Autodesk Inventor part; units mm, degrees
(part 3 of 4)
  line L1325 (-59.5167, -62.4834) -> (-59.6659, -62.6191)
  line L1326 (-59.6659, -62.6191) -> (-59.8276, -62.74)
  line L1327 (-59.8276, -62.74) -> (-60.0007, -62.8451)
  line L1328 (-60.0007, -62.8451) -> (-60.1844, -62.9336)
  line L1329 (-60.1844, -62.9336) -> (-60.3773, -63.0039)
  line L1330 (-60.3773, -63.0039) -> (-60.5785, -63.0559)
  line L1331 (-60.5785, -63.0559) -> (-60.7869, -63.0876)
  line L1332 (-60.7869, -63.0876) -> (-61.0017, -63.0986)
  line L1333 (-61.0017, -63.0986) -> (-61.2163, -63.0876)
  line L1334 (-61.2163, -63.0876) -> (-61.4249, -63.0559)
  line L1335 (-61.4249, -63.0559) -> (-61.6261, -63.0039)
  line L1336 (-61.6261, -63.0039) -> (-61.8191, -62.9336)
  line L1337 (-61.8191, -62.9336) -> (-62.0027, -62.8451)
  line L1338 (-62.0027, -62.8451) -> (-62.1758, -62.74)
  line L1339 (-62.1758, -62.74) -> (-62.3375, -62.6191)
  line L1340 (-62.3375, -62.6191) -> (-62.4865, -62.4834)
  line L1341 (-62.4865, -62.4834) -> (-62.6221, -62.3342)
  line L1342 (-62.6221, -62.3342) -> (-62.743, -62.1726)
  line L1343 (-62.743, -62.1726) -> (-62.8483, -61.9993)
  line L1344 (-62.8483, -61.9993) -> (-62.9366, -61.816)
  line L1345 (-62.9366, -61.816) -> (-63.0073, -61.6231)
  line L1346 (-63.0073, -61.6231) -> (-63.0589, -61.4216)
  line L1347 (-63.0589, -61.4216) -> (-63.0908, -61.2131)
  line L1348 (-63.0908, -61.2131) -> (-63.1017, -60.9985)
  line L1349 (59.4388, -47.6026) -> (59.4468, -47.4441)
  line L1350 (59.4468, -47.4441) -> (59.4705, -47.2901)
  line L1351 (59.4705, -47.2901) -> (59.5088, -47.1417)
  line L1352 (59.5088, -47.1417) -> (59.5608, -46.999)
  line L1353 (59.5608, -46.999) -> (59.7038, -46.7358)
  line L1354 (59.7038, -46.7358) -> (59.8929, -46.5064)
  line L1355 (59.8929, -46.5064) -> (60.1223, -46.3172)
  line L1356 (60.1223, -46.3172) -> (60.3855, -46.1743)
  line L1357 (60.3855, -46.1743) -> (60.5278, -46.1222)
  line L1358 (60.5278, -46.1222) -> (60.6767, -46.084)
  line L1359 (60.6767, -46.084) -> (60.8303, -46.0606)
  line L1360 (60.8303, -46.0606) -> (60.9888, -46.0527)
  line L1361 (60.9888, -46.0527) -> (61.1473, -46.0606)
  line L1362 (61.1473, -46.0606) -> (61.3013, -46.084)
  line L1363 (61.3013, -46.084) -> (61.4497, -46.1222)
  line L1364 (61.4497, -46.1222) -> (61.5924, -46.1743)
  line L1365 (61.5924, -46.1743) -> (61.8556, -46.3172)
  line L1366 (61.8556, -46.3172) -> (62.085, -46.5064)
  line L1367 (62.085, -46.5064) -> (62.2741, -46.7358)
  line L1368 (62.2741, -46.7358) -> (62.4171, -46.999)
  line L1369 (62.4171, -46.999) -> (62.4691, -47.1417)
  line L1370 (62.4691, -47.1417) -> (62.5074, -47.2901)
  line L1371 (62.5074, -47.2901) -> (62.5308, -47.4441)
  line L1372 (62.5308, -47.4441) -> (62.5391, -47.6026)
  line L1373 (62.5391, -47.6026) -> (62.5308, -47.7611)
  line L1374 (62.5308, -47.7611) -> (62.5074, -47.9147)
  line L1375 (62.5074, -47.9147) -> (62.4691, -48.0636)
  line L1376 (62.4691, -48.0636) -> (62.4171, -48.2058)
  line L1377 (62.4171, -48.2058) -> (62.2741, -48.469)
  line L1378 (62.2741, -48.469) -> (62.085, -48.6985)
  line L1379 (62.085, -48.6985) -> (61.8556, -48.888)
  line L1380 (61.8556, -48.888) -> (61.5924, -49.0306)
  line L1381 (61.5924, -49.0306) -> (61.4497, -49.083)
  line L1382 (61.4497, -49.083) -> (61.3013, -49.1209)
  line L1383 (61.3013, -49.1209) -> (61.1473, -49.1446)
  line L1384 (61.1473, -49.1446) -> (60.9888, -49.1526)
  line L1385 (60.9888, -49.1526) -> (60.8303, -49.1446)
  line L1386 (60.8303, -49.1446) -> (60.6767, -49.1209)
  line L1387 (60.6767, -49.1209) -> (60.5278, -49.083)
  line L1388 (60.5278, -49.083) -> (60.3855, -49.0306)
  line L1389 (60.3855, -49.0306) -> (60.1223, -48.888)
  line L1390 (60.1223, -48.888) -> (59.8929, -48.6985)
  line L1391 (59.8929, -48.6985) -> (59.7038, -48.469)
  line L1392 (59.7038, -48.469) -> (59.5608, -48.2058)
  line L1393 (59.5608, -48.2058) -> (59.5088, -48.0636)
  line L1394 (59.5088, -48.0636) -> (59.4705, -47.9147)
  line L1395 (59.4705, -47.9147) -> (59.4468, -47.7611)
  line L1396 (59.4468, -47.7611) -> (59.4388, -47.6026)
  line L1397 (-2.0682, 0) -> (2.0682, 0) construction
  line L1398 (0, 4.1364) -> (0, -4.1364) construction
  point P0 (0, 0)
  point P1 (0, 0)
  constraints: 1814 end point, 5 midpoint, 492 other
sketch "Sketch3" plane through (0, 0, 0) normal (0, 1, 0) x (-1, 0, 0)
  line L0 (-71.8987, -44.9902) -> (-71.8987, 45.0005) construction
  line L1 (71.8915, 29.9989) -> (71.8915, -29.9985) construction
  line L2 (-51.3449, 71.9911) -> (51.3515, 71.9911) construction
  line L3 (51.348, -71.9835) -> (-51.3468, -71.9835) construction
  line L4 (61.9413, 71.941) -> (-61.9413, 71.941)
  line L5 (-71.9413, 61.941) -> (-71.9413, -61.941)
  line L6 (-61.9413, -71.941) -> (61.9413, -71.941)
  line L7 (71.9413, -61.941) -> (71.9413, 61.941)
  line L8 (71.9413, 71.941) -> (-71.9413, -71.941) construction
  line L9 (-71.9413, 71.941) -> (71.9413, -71.941) construction
  arc A0 (-61.9413, 71.941) -> (-71.9413, 61.941) centre (-61.9413, 61.941) ccw
  arc A1 (71.9413, 61.941) -> (61.9413, 71.941) centre (61.9413, 61.941) ccw
  arc A2 (61.9413, -71.941) -> (71.9413, -61.941) centre (61.9413, -61.941) ccw
  arc A3 (-71.9413, -61.941) -> (-61.9413, -71.941) centre (-61.9413, -61.941) ccw
  line L10 (-41.1674, 56.1487) -> (-3.9986, 18.9801)
  line L11 (-3.9986, 18.9801) -> (-3.9986, 56.1578)
  line L12 (-3.9986, 56.1578) -> (-41.1674, 56.1487)
  line L13 (4.0012, 56.1578) -> (41.1357, 56.1578)
  line L14 (41.1357, 56.1578) -> (4.0012, 19.0231)
  line L15 (4.0012, 19.0231) -> (4.0012, 56.1578)
  line L16 (19.3996, 4.4418) -> (19.3996, -4.4032)
  line L17 (19.3996, -4.4032) -> (50.0055, -35.0091)
  line L18 (50.0055, -35.0091) -> (50.0055, 35.0476)
  line L19 (50.0055, 35.0476) -> (19.3996, 4.4418)
  line L20 (41.1109, -56.0179) -> (4.0012, -18.9084)
  line L21 (4.0012, -18.9084) -> (4.0012, -56.0179)
  line L22 (4.0012, -56.0179) -> (41.1109, -56.0179)
  line L23 (-3.9986, -56.0179) -> (-41.1514, -56.0179)
  line L24 (-41.1514, -56.0179) -> (-3.9986, -18.8653)
  line L25 (-3.9986, -18.8653) -> (-3.9986, -56.0179)
  line L26 (-50.007, -35.0077) -> (-19.4514, -4.0004)
  line L27 (-19.4514, -4.0004) -> (-19.4514, 4.453)
  line L28 (-19.4514, 4.453) -> (-50.007, 35.0084)
  line L29 (-50.007, 35.0084) -> (-50.007, -35.0077)
  point P0 (0, 0)
  point P1 (19.3996, 3.9996)
  dimension "d3" = 10
  constraints: 52 end point, 9 parallel, 8 point on circle, 8 point on line, 8 tangent, 6 perpendicular, 4 centre point, 3 equal radius, 2 midpoint, 1 collinear
  measures "d3" radius of A0
extrude "Extrusion1" add sketch "Sketch3" along normal blind 2
sketch "Sketch4" plane through (0, 0, 0) normal (0, -1, 0) x (1, 0, 0)
  line L0 (-41.1109, -56.0179) -> (-4.0012, -18.9084) projected
  line L1 (71.9413, 61.941) -> (71.9413, -61.941) projected
  line L2 (-61.9413, 71.941) -> (61.9413, 71.941) projected
  arc A0 (-61.9413, 71.941) -> (-71.9413, 61.941) centre (-61.9413, 61.941) ccw projected
  line L3 (-71.9413, -61.941) -> (-71.9413, 61.941) projected
  line L4 (61.9413, -71.941) -> (-61.9413, -71.941) projected
  circle A1 centre (-61.0413, 61.041) radius 2.1
  line L5 (0, 0) -> (-69.012, 69.0124) construction
  line L6 (-35.6206, 41.0655) -> (-43.7523, 49.1972)
  line L7 (-46.5807, 49.1972) -> (-49.197, 46.5809)
  line L8 (-49.197, 43.7525) -> (-41.0653, 35.6207)
  line L9 (-38.2369, 35.6207) -> (-35.6206, 38.237)
  line L10 (-34.2063, 39.6512) -> (-50.6112, 45.1667) construction
  line L11 (-45.1665, 50.6114) -> (-39.6511, 34.2065) construction
  arc A2 (-43.7523, 49.1972) -> (-46.5807, 49.1972) centre (-45.1665, 47.783) ccw
  arc A3 (-49.197, 46.5809) -> (-49.197, 43.7525) centre (-47.7828, 45.1667) ccw
  arc A4 (-41.0653, 35.6207) -> (-38.2369, 35.6207) centre (-39.6511, 37.035) ccw
  arc A5 (-35.6206, 38.237) -> (-35.6206, 41.0655) centre (-37.0348, 39.6512) ccw
  line L12 (14.1421, -14.1422) -> (-54.8699, 54.8702) construction
  line L13 (-21.4785, 26.9233) -> (-29.6102, 35.055)
  line L14 (-32.4386, 35.055) -> (-35.0549, 32.4388)
  line L15 (-35.0549, 29.6103) -> (-26.9232, 21.4786)
  line L16 (-24.0948, 21.4786) -> (-21.4785, 24.0949)
  line L17 (-20.0642, 25.5091) -> (-36.4691, 31.0245) construction
  line L18 (-31.0244, 36.4693) -> (-25.509, 20.0644) construction
  arc A6 (-29.6102, 35.055) -> (-32.4386, 35.055) centre (-31.0244, 33.6408) ccw
  arc A7 (-35.0549, 32.4388) -> (-35.0549, 29.6103) centre (-33.6407, 31.0245) ccw
  arc A8 (-26.9232, 21.4786) -> (-24.0948, 21.4786) centre (-25.509, 22.8928) ccw
  arc A9 (-21.4785, 24.0949) -> (-21.4785, 26.9233) centre (-22.8927, 25.5091) ccw
  line L19 (28.2842, -28.2843) -> (-40.7278, 40.728) construction
  line L20 (-7.3364, 12.7811) -> (-15.4681, 20.9129)
  line L21 (-18.2965, 20.9129) -> (-20.9128, 18.2966)
  line L22 (-20.9128, 15.4682) -> (-12.7811, 7.3364)
  line L23 (-9.9527, 7.3364) -> (-7.3364, 9.9527)
  line L24 (-5.9221, 11.3669) -> (-22.327, 16.8824) construction
  line L25 (-16.8823, 22.3271) -> (-11.3669, 5.9222) construction
  arc A10 (-15.4681, 20.9129) -> (-18.2965, 20.9129) centre (-16.8823, 19.4987) ccw
  arc A11 (-20.9128, 18.2966) -> (-20.9128, 15.4682) centre (-19.4986, 16.8824) ccw
  arc A12 (-12.7811, 7.3364) -> (-9.9527, 7.3364) centre (-11.3669, 8.7506) ccw
  arc A13 (-7.3364, 9.9527) -> (-7.3364, 12.7811) centre (-8.7506, 11.3669) ccw
  line L26 (-5.7083, 60.241) -> (5.6917, 60.241)
  line L27 (7.6917, 62.241) -> (7.6917, 65.941)
  line L28 (5.6917, 67.941) -> (-5.7083, 67.941)
  line L29 (-7.7083, 65.941) -> (-7.7083, 62.241)
  line L30 (-7.7083, 60.241) -> (7.6917, 67.941) construction
  line L31 (7.6917, 60.241) -> (-7.7083, 67.941) construction
  arc A14 (-5.7083, 67.941) -> (-7.7083, 65.941) centre (-5.7083, 65.941) ccw
  arc A15 (-7.7083, 62.241) -> (-5.7083, 60.241) centre (-5.7083, 62.241) ccw
  arc A16 (5.6917, 60.241) -> (7.6917, 62.241) centre (5.6917, 62.241) ccw
  arc A17 (7.6917, 65.941) -> (5.6917, 67.941) centre (5.6917, 65.941) ccw
  line L32 (-61.9413, 71.941) -> (0, 71.941) construction
  line L33 (0, 71.941) -> (0, -71.941) construction
  line L34 (14.2917, 60.241) -> (25.6917, 60.241)
  line L35 (27.6917, 62.241) -> (27.6917, 65.941)
  line L36 (25.6917, 67.941) -> (14.2917, 67.941)
  line L37 (12.2917, 65.941) -> (12.2917, 62.241)
  line L38 (12.2917, 60.241) -> (27.6917, 67.941) construction
  line L39 (27.6917, 60.241) -> (12.2917, 67.941) construction
  arc A18 (14.2917, 67.941) -> (12.2917, 65.941) centre (14.2917, 65.941) ccw
  arc A19 (12.2917, 62.241) -> (14.2917, 60.241) centre (14.2917, 62.241) ccw
  arc A20 (25.6917, 60.241) -> (27.6917, 62.241) centre (25.6917, 62.241) ccw
  arc A21 (27.6917, 65.941) -> (25.6917, 67.941) centre (25.6917, 65.941) ccw
  line L40 (34.2917, 60.241) -> (45.6917, 60.241)
  line L41 (47.6917, 62.241) -> (47.6917, 65.941)
  line L42 (45.6917, 67.941) -> (34.2917, 67.941)
  line L43 (32.2917, 65.941) -> (32.2917, 62.241)
  line L44 (32.2917, 60.241) -> (47.6917, 67.941) construction
  line L45 (47.6917, 60.241) -> (32.2917, 67.941) construction
  arc A22 (34.2917, 67.941) -> (32.2917, 65.941) centre (34.2917, 65.941) ccw
  arc A23 (32.2917, 62.241) -> (34.2917, 60.241) centre (34.2917, 62.241) ccw
  arc A24 (45.6917, 60.241) -> (47.6917, 62.241) centre (45.6917, 62.241) ccw
  arc A25 (47.6917, 65.941) -> (45.6917, 67.941) centre (45.6917, 65.941) ccw
  line L46 (-25.7083, 60.241) -> (-14.3083, 60.241)
  line L47 (-12.3083, 62.241) -> (-12.3083, 65.941)
  line L48 (-14.3083, 67.941) -> (-25.7083, 67.941)
  line L49 (-27.7083, 65.941) -> (-27.7083, 62.241)
  line L50 (-27.7083, 60.241) -> (-12.3083, 67.941) construction
  line L51 (-12.3083, 60.241) -> (-27.7083, 67.941) construction
  arc A26 (-25.7083, 67.941) -> (-27.7083, 65.941) centre (-25.7083, 65.941) ccw
  arc A27 (-27.7083, 62.241) -> (-25.7083, 60.241) centre (-25.7083, 62.241) ccw
  arc A28 (-14.3083, 60.241) -> (-12.3083, 62.241) centre (-14.3083, 62.241) ccw
  arc A29 (-12.3083, 65.941) -> (-14.3083, 67.941) centre (-14.3083, 65.941) ccw
  line L52 (-5.7083, 60.241) -> (5.6917, 60.241)
  line L53 (7.6917, 62.241) -> (7.6917, 65.941)
  line L54 (5.6917, 67.941) -> (-5.7083, 67.941)
  line L55 (-7.7083, 65.941) -> (-7.7083, 62.241)
  line L56 (-7.7083, 60.241) -> (7.6917, 67.941) construction
  line L57 (7.6917, 60.241) -> (-7.7083, 67.941) construction
  arc A30 (-5.7083, 67.941) -> (-7.7083, 65.941) centre (-5.7083, 65.941) ccw
  arc A31 (-7.7083, 62.241) -> (-5.7083, 60.241) centre (-5.7083, 62.241) ccw
  arc A32 (5.6917, 60.241) -> (7.6917, 62.241) centre (5.6917, 62.241) ccw
  arc A33 (7.6917, 65.941) -> (5.6917, 67.941) centre (5.6917, 65.941) ccw
  line L58 (14.2917, 60.241) -> (25.6917, 60.241)
  line L59 (27.6917, 62.241) -> (27.6917, 65.941)
  line L60 (25.6917, 67.941) -> (14.2917, 67.941)
  line L61 (12.2917, 65.941) -> (12.2917, 62.241)
  line L62 (12.2917, 60.241) -> (27.6917, 67.941) construction
  line L63 (27.6917, 60.241) -> (12.2917, 67.941) construction
  arc A34 (14.2917, 67.941) -> (12.2917, 65.941) centre (14.2917, 65.941) ccw
  arc A35 (12.2917, 62.241) -> (14.2917, 60.241) centre (14.2917, 62.241) ccw
  arc A36 (25.6917, 60.241) -> (27.6917, 62.241) centre (25.6917, 62.241) ccw
  arc A37 (27.6917, 65.941) -> (25.6917, 67.941) centre (25.6917, 65.941) ccw
  line L64 (-45.7083, 60.241) -> (-34.3083, 60.241)
  line L65 (-32.3083, 62.241) -> (-32.3083, 65.941)
  line L66 (-34.3083, 67.941) -> (-45.7083, 67.941)
  line L67 (-47.7083, 65.941) -> (-47.7083, 62.241)
  line L68 (-47.7083, 60.241) -> (-32.3083, 67.941) construction
  line L69 (-32.3083, 60.241) -> (-47.7083, 67.941) construction
  arc A38 (-45.7083, 67.941) -> (-47.7083, 65.941) centre (-45.7083, 65.941) ccw
  arc A39 (-47.7083, 62.241) -> (-45.7083, 60.241) centre (-45.7083, 62.241) ccw
  arc A40 (-34.3083, 60.241) -> (-32.3083, 62.241) centre (-34.3083, 62.241) ccw
  arc A41 (-32.3083, 65.941) -> (-34.3083, 67.941) centre (-34.3083, 65.941) ccw
  line L70 (-25.7083, 60.241) -> (-14.3083, 60.241)
  line L71 (-12.3083, 62.241) -> (-12.3083, 65.941)
  line L72 (-14.3083, 67.941) -> (-25.7083, 67.941)
  line L73 (-27.7083, 65.941) -> (-27.7083, 62.241)
  line L74 (-27.7083, 60.241) -> (-12.3083, 67.941) construction
  line L75 (-12.3083, 60.241) -> (-27.7083, 67.941) construction
  arc A42 (-25.7083, 67.941) -> (-27.7083, 65.941) centre (-25.7083, 65.941) ccw
  arc A43 (-27.7083, 62.241) -> (-25.7083, 60.241) centre (-25.7083, 62.241) ccw
  arc A44 (-14.3083, 60.241) -> (-12.3083, 62.241) centre (-14.3083, 62.241) ccw
  arc A45 (-12.3083, 65.941) -> (-14.3083, 67.941) centre (-14.3083, 65.941) ccw
  line L76 (-5.7083, 60.241) -> (5.6917, 60.241)
  line L77 (7.6917, 62.241) -> (7.6917, 65.941)
  line L78 (5.6917, 67.941) -> (-5.7083, 67.941)
  line L79 (-7.7083, 65.941) -> (-7.7083, 62.241)
  line L80 (-7.7083, 60.241) -> (7.6917, 67.941) construction
  line L81 (7.6917, 60.241) -> (-7.7083, 67.941) construction
  arc A46 (-5.7083, 67.941) -> (-7.7083, 65.941) centre (-5.7083, 65.941) ccw
  arc A47 (-7.7083, 62.241) -> (-5.7083, 60.241) centre (-5.7083, 62.241) ccw
  arc A48 (5.6917, 60.241) -> (7.6917, 62.241) centre (5.6917, 62.241) ccw
  arc A49 (7.6917, 65.941) -> (5.6917, 67.941) centre (5.6917, 65.941) ccw
  line L82 (-71.9413, 0) -> (71.9413, 0) construction
  line L83 (-5.7083, -60.241) -> (5.6917, -60.241)
  line L84 (7.6917, -62.241) -> (7.6917, -65.941)
  line L85 (5.6917, -67.941) -> (-5.7083, -67.941)
  line L86 (-7.7083, -65.941) -> (-7.7083, -62.241)
  line L87 (-7.7083, -60.241) -> (7.6917, -67.941) construction
  line L88 (7.6917, -60.241) -> (-7.7083, -67.941) construction
  arc A50 (-7.7083, -65.941) -> (-5.7083, -67.941) centre (-5.7083, -65.941) ccw
  arc A51 (-5.7083, -60.241) -> (-7.7083, -62.241) centre (-5.7083, -62.241) ccw
  arc A52 (7.6917, -62.241) -> (5.6917, -60.241) centre (5.6917, -62.241) ccw
  arc A53 (5.6917, -67.941) -> (7.6917, -65.941) centre (5.6917, -65.941) ccw
  line L89 (0, -71.941) -> (0, 71.941) construction
  line L90 (27.6917, -62.241) -> (27.6917, -65.941)
  line L91 (25.6917, -67.941) -> (14.2917, -67.941)
  line L92 (14.2917, -60.241) -> (25.6917, -60.241)
  arc A54 (25.6917, -67.941) -> (27.6917, -65.941) centre (25.6917, -65.941) ccw
  line L93 (12.2917, -60.241) -> (27.6917, -67.941) construction
  line L94 (27.6917, -60.241) -> (12.2917, -67.941) construction
  arc A55 (14.2917, -60.241) -> (12.2917, -62.241) centre (14.2917, -62.241) ccw
  arc A56 (12.2917, -65.941) -> (14.2917, -67.941) centre (14.2917, -65.941) ccw
  line L95 (12.2917, -65.941) -> (12.2917, -62.241)
  arc A57 (27.6917, -62.241) -> (25.6917, -60.241) centre (25.6917, -62.241) ccw
  line L96 (47.6917, -62.241) -> (47.6917, -65.941)
  line L97 (45.6917, -67.941) -> (34.2917, -67.941)
  line L98 (34.2917, -60.241) -> (45.6917, -60.241)
  arc A58 (45.6917, -67.941) -> (47.6917, -65.941) centre (45.6917, -65.941) ccw
  line L99 (32.2917, -60.241) -> (47.6917, -67.941) construction
  line L100 (47.6917, -60.241) -> (32.2917, -67.941) construction
  arc A59 (34.2917, -60.241) -> (32.2917, -62.241) centre (34.2917, -62.241) ccw
  arc A60 (32.2917, -65.941) -> (34.2917, -67.941) centre (34.2917, -65.941) ccw
  line L101 (32.2917, -65.941) -> (32.2917, -62.241)
  arc A61 (47.6917, -62.241) -> (45.6917, -60.241) centre (45.6917, -62.241) ccw
  line L102 (-12.3083, -62.241) -> (-12.3083, -65.941)
  line L103 (-14.3083, -67.941) -> (-25.7083, -67.941)
  line L104 (-25.7083, -60.241) -> (-14.3083, -60.241)
  arc A62 (-14.3083, -67.941) -> (-12.3083, -65.941) centre (-14.3083, -65.941) ccw
  line L105 (-27.7083, -60.241) -> (-12.3083, -67.941) construction
  line L106 (-12.3083, -60.241) -> (-27.7083, -67.941) construction
  arc A63 (-25.7083, -60.241) -> (-27.7083, -62.241) centre (-25.7083, -62.241) ccw
  arc A64 (-27.7083, -65.941) -> (-25.7083, -67.941) centre (-25.7083, -65.941) ccw
  line L107 (-27.7083, -65.941) -> (-27.7083, -62.241)
  arc A65 (-12.3083, -62.241) -> (-14.3083, -60.241) centre (-14.3083, -62.241) ccw
  line L108 (7.6917, -62.241) -> (7.6917, -65.941)
  line L109 (5.6917, -67.941) -> (-5.7083, -67.941)
  line L110 (-5.7083, -60.241) -> (5.6917, -60.241)
  arc A66 (5.6917, -67.941) -> (7.6917, -65.941) centre (5.6917, -65.941) ccw
  line L111 (-7.7083, -60.241) -> (7.6917, -67.941) construction
  line L112 (7.6917, -60.241) -> (-7.7083, -67.941) construction
  arc A67 (-5.7083, -60.241) -> (-7.7083, -62.241) centre (-5.7083, -62.241) ccw
  arc A68 (-7.7083, -65.941) -> (-5.7083, -67.941) centre (-5.7083, -65.941) ccw
  line L113 (-7.7083, -65.941) -> (-7.7083, -62.241)
  arc A69 (7.6917, -62.241) -> (5.6917, -60.241) centre (5.6917, -62.241) ccw
  line L114 (27.6917, -62.241) -> (27.6917, -65.941)
  line L115 (25.6917, -67.941) -> (14.2917, -67.941)
  line L116 (14.2917, -60.241) -> (25.6917, -60.241)
  arc A70 (25.6917, -67.941) -> (27.6917, -65.941) centre (25.6917, -65.941) ccw
  line L117 (12.2917, -60.241) -> (27.6917, -67.941) construction
  line L118 (27.6917, -60.241) -> (12.2917, -67.941) construction
  arc A71 (14.2917, -60.241) -> (12.2917, -62.241) centre (14.2917, -62.241) ccw
  arc A72 (12.2917, -65.941) -> (14.2917, -67.941) centre (14.2917, -65.941) ccw
  line L119 (12.2917, -65.941) -> (12.2917, -62.241)
  arc A73 (27.6917, -62.241) -> (25.6917, -60.241) centre (25.6917, -62.241) ccw
  line L120 (-32.3083, -62.241) -> (-32.3083, -65.941)
  line L121 (-34.3083, -67.941) -> (-45.7083, -67.941)
  line L122 (-45.7083, -60.241) -> (-34.3083, -60.241)
  arc A74 (-34.3083, -67.941) -> (-32.3083, -65.941) centre (-34.3083, -65.941) ccw
  line L123 (-47.7083, -60.241) -> (-32.3083, -67.941) construction
  line L124 (-32.3083, -60.241) -> (-47.7083, -67.941) construction
  arc A75 (-45.7083, -60.241) -> (-47.7083, -62.241) centre (-45.7083, -62.241) ccw
  arc A76 (-47.7083, -65.941) -> (-45.7083, -67.941) centre (-45.7083, -65.941) ccw
  line L125 (-47.7083, -65.941) -> (-47.7083, -62.241)
  arc A77 (-32.3083, -62.241) -> (-34.3083, -60.241) centre (-34.3083, -62.241) ccw
  line L126 (-12.3083, -62.241) -> (-12.3083, -65.941)
  line L127 (-14.3083, -67.941) -> (-25.7083, -67.941)
  line L128 (-25.7083, -60.241) -> (-14.3083, -60.241)
  arc A78 (-14.3083, -67.941) -> (-12.3083, -65.941) centre (-14.3083, -65.941) ccw
  line L129 (-27.7083, -60.241) -> (-12.3083, -67.941) construction
  line L130 (-12.3083, -60.241) -> (-27.7083, -67.941) construction
  arc A79 (-25.7083, -60.241) -> (-27.7083, -62.241) centre (-25.7083, -62.241) ccw
  arc A80 (-27.7083, -65.941) -> (-25.7083, -67.941) centre (-25.7083, -65.941) ccw
  line L131 (-27.7083, -65.941) -> (-27.7083, -62.241)
  arc A81 (-12.3083, -62.241) -> (-14.3083, -60.241) centre (-14.3083, -62.241) ccw
  line L132 (7.6917, -62.241) -> (7.6917, -65.941)
  line L133 (5.6917, -67.941) -> (-5.7083, -67.941)
  line L134 (-5.7083, -60.241) -> (5.6917, -60.241)
  arc A82 (5.6917, -67.941) -> (7.6917, -65.941) centre (5.6917, -65.941) ccw
  line L135 (-7.7083, -60.241) -> (7.6917, -67.941) construction
  line L136 (7.6917, -60.241) -> (-7.7083, -67.941) construction
  arc A83 (-5.7083, -60.241) -> (-7.7083, -62.241) centre (-5.7083, -62.241) ccw
  arc A84 (-7.7083, -65.941) -> (-5.7083, -67.941) centre (-5.7083, -65.941) ccw
  line L137 (-7.7083, -65.941) -> (-7.7083, -62.241)
  arc A85 (7.6917, -62.241) -> (5.6917, -60.241) centre (5.6917, -62.241) ccw
  line L138 (0, 0) -> (-51.9765, -51.9763) construction
  line L139 (0, 0) -> (-69.012, -69.0124) construction
  line L140 (-35.6206, -41.0655) -> (-43.7523, -49.1972)
  line L141 (-46.5807, -49.1972) -> (-49.197, -46.5809)
  line L142 (-49.197, -43.7525) -> (-41.0653, -35.6207)
  line L143 (-38.2369, -35.6207) -> (-35.6206, -38.237)
  line L144 (-34.2063, -39.6512) -> (-50.6112, -45.1667) construction
  line L145 (-45.1665, -50.6114) -> (-39.6511, -34.2065) construction
  arc A86 (-46.5807, -49.1972) -> (-43.7523, -49.1972) centre (-45.1665, -47.783) ccw
  arc A87 (-49.197, -43.7525) -> (-49.197, -46.5809) centre (-47.7828, -45.1667) ccw
  arc A88 (-38.2369, -35.6207) -> (-41.0653, -35.6207) centre (-39.6511, -37.035) ccw
  arc A89 (-35.6206, -41.0655) -> (-35.6206, -38.237) centre (-37.0348, -39.6512) ccw
  line L146 (-32.4386, -35.055) -> (-35.0549, -32.4388)
  arc A90 (-35.0549, -29.6103) -> (-35.0549, -32.4388) centre (-33.6407, -31.0245) ccw
  line L147 (-21.4785, -26.9233) -> (-29.6102, -35.055)
  arc A91 (-24.0948, -21.4786) -> (-26.9232, -21.4786) centre (-25.509, -22.8928) ccw
  line L148 (-35.0549, -29.6103) -> (-26.9232, -21.4786)
  line L149 (-31.0244, -36.4693) -> (-25.509, -20.0644) construction
  line L150 (-24.0948, -21.4786) -> (-21.4785, -24.0949)
  line L151 (-20.0642, -25.5091) -> (-36.4691, -31.0245) construction
  line L152 (14.1421, 14.1422) -> (-54.8699, -54.8702) construction
  arc A92 (-21.4785, -26.9233) -> (-21.4785, -24.0949) centre (-22.8927, -25.5091) ccw
  arc A93 (-32.4386, -35.055) -> (-29.6102, -35.055) centre (-31.0244, -33.6408) ccw
  line L153 (-18.2965, -20.9129) -> (-20.9128, -18.2966)
  arc A94 (-20.9128, -15.4682) -> (-20.9128, -18.2966) centre (-19.4986, -16.8824) ccw
  line L154 (-7.3364, -12.7811) -> (-15.4681, -20.9129)
  arc A95 (-9.9527, -7.3364) -> (-12.7811, -7.3364) centre (-11.3669, -8.7506) ccw
  line L155 (-20.9128, -15.4682) -> (-12.7811, -7.3364)
  line L156 (-16.8823, -22.3271) -> (-11.3669, -5.9222) construction
  line L157 (-9.9527, -7.3364) -> (-7.3364, -9.9527)
  line L158 (-5.9221, -11.3669) -> (-22.327, -16.8824) construction
  line L159 (28.2842, 28.2843) -> (-40.7278, -40.728) construction
  arc A96 (-7.3364, -12.7811) -> (-7.3364, -9.9527) centre (-8.7506, -11.3669) ccw
  arc A97 (-18.2965, -20.9129) -> (-15.4681, -20.9129) centre (-16.8823, -19.4987) ccw
  line L160 (35.6206, 41.0655) -> (43.7523, 49.1972)
  line L161 (46.5807, 49.1972) -> (49.197, 46.5809)
  line L162 (49.197, 43.7525) -> (41.0653, 35.6207)
  line L163 (38.2369, 35.6207) -> (35.6206, 38.237)
  line L164 (34.2063, 39.6512) -> (50.6112, 45.1667) construction
  line L165 (45.1665, 50.6114) -> (39.6511, 34.2065) construction
  arc A98 (46.5807, 49.1972) -> (43.7523, 49.1972) centre (45.1665, 47.783) ccw
  arc A99 (49.197, 43.7525) -> (49.197, 46.5809) centre (47.7828, 45.1667) ccw
  arc A100 (38.2369, 35.6207) -> (41.0653, 35.6207) centre (39.6511, 37.035) ccw
  arc A101 (35.6206, 41.0655) -> (35.6206, 38.237) centre (37.0348, 39.6512) ccw
  line L166 (32.4386, 35.055) -> (35.0549, 32.4388)
  arc A102 (35.0549, 29.6103) -> (35.0549, 32.4388) centre (33.6407, 31.0245) ccw
  line L167 (21.4785, 26.9233) -> (29.6102, 35.055)
  arc A103 (24.0948, 21.4786) -> (26.9232, 21.4786) centre (25.509, 22.8928) ccw
  line L168 (35.0549, 29.6103) -> (26.9232, 21.4786)
  line L169 (31.0244, 36.4693) -> (25.509, 20.0644) construction
  line L170 (24.0948, 21.4786) -> (21.4785, 24.0949)
  line L171 (20.0642, 25.5091) -> (36.4691, 31.0245) construction
  arc A104 (21.4785, 26.9233) -> (21.4785, 24.0949) centre (22.8927, 25.5091) ccw
  arc A105 (32.4386, 35.055) -> (29.6102, 35.055) centre (31.0244, 33.6408) ccw
  line L172 (18.2965, 20.9129) -> (20.9128, 18.2966)
  arc A106 (20.9128, 15.4682) -> (20.9128, 18.2966) centre (19.4986, 16.8824) ccw
  line L173 (7.3364, 12.7811) -> (15.4681, 20.9129)
  arc A107 (9.9527, 7.3364) -> (12.7811, 7.3364) centre (11.3669, 8.7506) ccw
  line L174 (20.9128, 15.4682) -> (12.7811, 7.3364)
  line L175 (16.8823, 22.3271) -> (11.3669, 5.9222) construction
  line L176 (9.9527, 7.3364) -> (7.3364, 9.9527)
  line L177 (5.9221, 11.3669) -> (22.327, 16.8824) construction
  arc A108 (7.3364, 12.7811) -> (7.3364, 9.9527) centre (8.7506, 11.3669) ccw
  arc A109 (18.2965, 20.9129) -> (15.4681, 20.9129) centre (16.8823, 19.4987) ccw
  line L178 (71.9413, 0) -> (-71.9413, 0) construction
  line L179 (0, 0) -> (51.9765, -51.9763) construction
  arc A110 (12.7811, -7.3364) -> (9.9527, -7.3364) centre (11.3669, -8.7506) ccw
  line L180 (9.9527, -7.3364) -> (7.3364, -9.9527)
  line L181 (7.3364, -12.7811) -> (15.4681, -20.9129)
  line L182 (16.8823, -22.3271) -> (11.3669, -5.9222) construction
  line L183 (20.9128, -15.4682) -> (12.7811, -7.3364)
  line L184 (5.9221, -11.3669) -> (22.327, -16.8824) construction
  line L185 (0, 0) -> (69.012, -69.0124) construction
  arc A111 (7.3364, -9.9527) -> (7.3364, -12.7811) centre (8.7506, -11.3669) ccw
  line L186 (24.0948, -21.4786) -> (21.4785, -24.0949)
  arc A112 (26.9232, -21.4786) -> (24.0948, -21.4786) centre (25.509, -22.8928) ccw
  arc A113 (21.4785, -24.0949) -> (21.4785, -26.9233) centre (22.8927, -25.5091) ccw
  line L187 (31.0244, -36.4693) -> (25.509, -20.0644) construction
  arc A114 (20.9128, -18.2966) -> (20.9128, -15.4682) centre (19.4986, -16.8824) ccw
  line L188 (18.2965, -20.9129) -> (20.9128, -18.2966)
  arc A115 (15.4681, -20.9129) -> (18.2965, -20.9129) centre (16.8823, -19.4987) ccw
  line L189 (21.4785, -26.9233) -> (29.6102, -35.055)
  arc A116 (29.6102, -35.055) -> (32.4386, -35.055) centre (31.0244, -33.6408) ccw
  line L190 (35.0549, -29.6103) -> (26.9232, -21.4786)
  line L191 (20.0642, -25.5091) -> (36.4691, -31.0245) construction
  arc A117 (35.0549, -32.4388) -> (35.0549, -29.6103) centre (33.6407, -31.0245) ccw
  line L192 (32.4386, -35.055) -> (35.0549, -32.4388)
  line L193 (49.197, -43.7525) -> (41.0653, -35.6207)
  line L194 (38.2369, -35.6207) -> (35.6206, -38.237)
  line L195 (45.1665, -50.6114) -> (39.6511, -34.2065) construction
  line L196 (35.6206, -41.0655) -> (43.7523, -49.1972)
  arc A118 (41.0653, -35.6207) -> (38.2369, -35.6207) centre (39.6511, -37.035) ccw
  arc A119 (35.6206, -38.237) -> (35.6206, -41.0655) centre (37.0348, -39.6512) ccw
  line L197 (46.5807, -49.1972) -> (49.197, -46.5809)
  arc A120 (43.7523, -49.1972) -> (46.5807, -49.1972) centre (45.1665, -47.783) ccw
  arc A121 (49.197, -46.5809) -> (49.197, -43.7525) centre (47.7828, -45.1667) ccw
  line L198 (-19.3996, 4.4418) -> (-19.3996, -4.4032) projected
  arc A122 (71.9413, 61.941) -> (61.9413, 71.941) centre (61.9413, 61.941) ccw projected
  circle A123 centre (61.0413, 61.041) radius 2.1
  circle A124 centre (-61.0413, -61.041) radius 2.1
  line L199 (14.1421, 14.1422) -> (-54.8699, -54.8702) construction
  circle A125 centre (61.0413, -61.041) radius 2.1
  circle A126 centre (-10.4996, 0) radius 2.5
  circle A127 centre (10.4996, 0) radius 2.5
  line L200 (-0.8722, -4.1286) -> (0.8722, -4.1286)
  line L201 (2.0722, -2.9286) -> (2.0722, 2.9286)
  line L202 (0.8722, 4.1286) -> (-0.8722, 4.1286)
  line L203 (-2.0722, 2.9286) -> (-2.0722, -2.9286)
  line L204 (-2.0722, -4.1286) -> (2.0722, 4.1286) construction
  line L205 (2.0722, -4.1286) -> (-2.0722, 4.1286) construction
  arc A128 (-0.8722, 4.1286) -> (-2.0722, 2.9286) centre (-0.8722, 2.9286) ccw
  arc A129 (2.0722, 2.9286) -> (0.8722, 4.1286) centre (0.8722, 2.9286) ccw
  arc A130 (0.8722, -4.1286) -> (2.0722, -2.9286) centre (0.8722, -2.9286) ccw
  arc A131 (-2.0722, -2.9286) -> (-0.8722, -4.1286) centre (-0.8722, -2.9286) ccw
  line L206 (-0.8722, 8.2814) -> (0.8722, 8.2814)
  line L207 (2.0722, 9.4814) -> (2.0722, 15.3386)
  line L208 (0.8722, 16.5386) -> (-0.8722, 16.5386)
  line L209 (-2.0722, 15.3386) -> (-2.0722, 9.4814)
  line L210 (-2.0722, 8.2814) -> (2.0722, 16.5386) construction
  line L211 (2.0722, 8.2814) -> (-2.0722, 16.5386) construction
  arc A132 (-0.8722, 16.5386) -> (-2.0722, 15.3386) centre (-0.8722, 15.3386) ccw
  arc A133 (2.0722, 15.3386) -> (0.8722, 16.5386) centre (0.8722, 15.3386) ccw
  arc A134 (0.8722, 8.2814) -> (2.0722, 9.4814) centre (0.8722, 9.4814) ccw
  arc A135 (-2.0722, 9.4814) -> (-0.8722, 8.2814) centre (-0.8722, 9.4814) ccw
  line L212 (-0.8722, 20.6914) -> (0.8722, 20.6914)
  line L213 (2.0722, 21.8914) -> (2.0722, 27.7486)
  line L214 (0.8722, 28.9486) -> (-0.8722, 28.9486)
  line L215 (-2.0722, 27.7486) -> (-2.0722, 21.8914)
  line L216 (-2.0722, 20.6914) -> (2.0722, 28.9486) construction
  line L217 (2.0722, 20.6914) -> (-2.0722, 28.9486) construction
  arc A136 (-0.8722, 28.9486) -> (-2.0722, 27.7486) centre (-0.8722, 27.7486) ccw
  arc A137 (2.0722, 27.7486) -> (0.8722, 28.9486) centre (0.8722, 27.7486) ccw
  arc A138 (0.8722, 20.6914) -> (2.0722, 21.8914) centre (0.8722, 21.8914) ccw
  arc A139 (-2.0722, 21.8914) -> (-0.8722, 20.6914) centre (-0.8722, 21.8914) ccw
  line L218 (-0.8722, 33.1014) -> (0.8722, 33.1014)
  line L219 (2.0722, 34.3014) -> (2.0722, 40.1586)
  line L220 (0.8722, 41.3586) -> (-0.8722, 41.3586)
  line L221 (-2.0722, 40.1586) -> (-2.0722, 34.3014)
  line L222 (-2.0722, 33.1014) -> (2.0722, 41.3586) construction
  line L223 (2.0722, 33.1014) -> (-2.0722, 41.3586) construction
  arc A140 (-0.8722, 41.3586) -> (-2.0722, 40.1586) centre (-0.8722, 40.1586) ccw
  arc A141 (2.0722, 40.1586) -> (0.8722, 41.3586) centre (0.8722, 40.1586) ccw
  arc A142 (0.8722, 33.1014) -> (2.0722, 34.3014) centre (0.8722, 34.3014) ccw
  arc A143 (-2.0722, 34.3014) -> (-0.8722, 33.1014) centre (-0.8722, 34.3014) ccw
  line L224 (-0.8722, 45.5114) -> (0.8722, 45.5114)
  line L225 (2.0722, 46.7114) -> (2.0722, 52.5686)
  line L226 (0.8722, 53.7686) -> (-0.8722, 53.7686)
  line L227 (-2.0722, 52.5686) -> (-2.0722, 46.7114)
  line L228 (-2.0722, 45.5114) -> (2.0722, 53.7686) construction
  line L229 (2.0722, 45.5114) -> (-2.0722, 53.7686) construction
  arc A144 (-0.8722, 53.7686) -> (-2.0722, 52.5686) centre (-0.8722, 52.5686) ccw
  arc A145 (2.0722, 52.5686) -> (0.8722, 53.7686) centre (0.8722, 52.5686) ccw
  arc A146 (0.8722, 45.5114) -> (2.0722, 46.7114) centre (0.8722, 46.7114) ccw
  arc A147 (-2.0722, 46.7114) -> (-0.8722, 45.5114) centre (-0.8722, 46.7114) ccw
  line L230 (-0.8722, -16.5386) -> (0.8722, -16.5386)
  line L231 (2.0722, -15.3386) -> (2.0722, -9.4814)
  line L232 (0.8722, -8.2814) -> (-0.8722, -8.2814)
  line L233 (-2.0722, -9.4814) -> (-2.0722, -15.3386)
  line L234 (-2.0722, -16.5386) -> (2.0722, -8.2814) construction
  line L235 (2.0722, -16.5386) -> (-2.0722, -8.2814) construction
  arc A148 (-0.8722, -8.2814) -> (-2.0722, -9.4814) centre (-0.8722, -9.4814) ccw
  arc A149 (2.0722, -9.4814) -> (0.8722, -8.2814) centre (0.8722, -9.4814) ccw
  arc A150 (0.8722, -16.5386) -> (2.0722, -15.3386) centre (0.8722, -15.3386) ccw
  arc A151 (-2.0722, -15.3386) -> (-0.8722, -16.5386) centre (-0.8722, -15.3386) ccw
  line L236 (-0.8722, -4.1286) -> (0.8722, -4.1286)
  line L237 (2.0722, -2.9286) -> (2.0722, 2.9286)
  line L238 (0.8722, 4.1286) -> (-0.8722, 4.1286)
  line L239 (-2.0722, 2.9286) -> (-2.0722, -2.9286)
  line L240 (-2.0722, -4.1286) -> (2.0722, 4.1286) construction
  line L241 (2.0722, -4.1286) -> (-2.0722, 4.1286) construction
  arc A152 (-0.8722, 4.1286) -> (-2.0722, 2.9286) centre (-0.8722, 2.9286) ccw
  arc A153 (2.0722, 2.9286) -> (0.8722, 4.1286) centre (0.8722, 2.9286) ccw
  arc A154 (0.8722, -4.1286) -> (2.0722, -2.9286) centre (0.8722, -2.9286) ccw
  arc A155 (-2.0722, -2.9286) -> (-0.8722, -4.1286) centre (-0.8722, -2.9286) ccw
  line L242 (-0.8722, 8.2814) -> (0.8722, 8.2814)
  line L243 (2.0722, 9.4814) -> (2.0722, 15.3386)
  line L244 (0.8722, 16.5386) -> (-0.8722, 16.5386)
  line L245 (-2.0722, 15.3386) -> (-2.0722, 9.4814)
  line L246 (-2.0722, 8.2814) -> (2.0722, 16.5386) construction
  line L247 (2.0722, 8.2814) -> (-2.0722, 16.5386) construction
  arc A156 (-0.8722, 16.5386) -> (-2.0722, 15.3386) centre (-0.8722, 15.3386) ccw
  arc A157 (2.0722, 15.3386) -> (0.8722, 16.5386) centre (0.8722, 15.3386) ccw
  arc A158 (0.8722, 8.2814) -> (2.0722, 9.4814) centre (0.8722, 9.4814) ccw
  arc A159 (-2.0722, 9.4814) -> (-0.8722, 8.2814) centre (-0.8722, 9.4814) ccw
  line L248 (-0.8722, 20.6914) -> (0.8722, 20.6914)
  line L249 (2.0722, 21.8914) -> (2.0722, 27.7486)
  line L250 (0.8722, 28.9486) -> (-0.8722, 28.9486)
  line L251 (-2.0722, 27.7486) -> (-2.0722, 21.8914)
  line L252 (-2.0722, 20.6914) -> (2.0722, 28.9486) construction
  line L253 (2.0722, 20.6914) -> (-2.0722, 28.9486) construction
  arc A160 (-0.8722, 28.9486) -> (-2.0722, 27.7486) centre (-0.8722, 27.7486) ccw
  arc A161 (2.0722, 27.7486) -> (0.8722, 28.9486) centre (0.8722, 27.7486) ccw
  arc A162 (0.8722, 20.6914) -> (2.0722, 21.8914) centre (0.8722, 21.8914) ccw
  arc A163 (-2.0722, 21.8914) -> (-0.8722, 20.6914) centre (-0.8722, 21.8914) ccw
  line L254 (-0.8722, 33.1014) -> (0.8722, 33.1014)
  line L255 (2.0722, 34.3014) -> (2.0722, 40.1586)
  line L256 (0.8722, 41.3586) -> (-0.8722, 41.3586)
  line L257 (-2.0722, 40.1586) -> (-2.0722, 34.3014)
  line L258 (-2.0722, 33.1014) -> (2.0722, 41.3586) construction
  line L259 (2.0722, 33.1014) -> (-2.0722, 41.3586) construction
  arc A164 (-0.8722, 41.3586) -> (-2.0722, 40.1586) centre (-0.8722, 40.1586) ccw
  arc A165 (2.0722, 40.1586) -> (0.8722, 41.3586) centre (0.8722, 40.1586) ccw
  arc A166 (0.8722, 33.1014) -> (2.0722, 34.3014) centre (0.8722, 34.3014) ccw
  arc A167 (-2.0722, 34.3014) -> (-0.8722, 33.1014) centre (-0.8722, 34.3014) ccw
  line L260 (-0.8722, -28.9486) -> (0.8722, -28.9486)
  line L261 (2.0722, -27.7486) -> (2.0722, -21.8914)
  line L262 (0.8722, -20.6914) -> (-0.8722, -20.6914)
  line L263 (-2.0722, -21.8914) -> (-2.0722, -27.7486)
  line L264 (-2.0722, -28.9486) -> (2.0722, -20.6914) construction
  line L265 (2.0722, -28.9486) -> (-2.0722, -20.6914) construction
  arc A168 (-0.8722, -20.6914) -> (-2.0722, -21.8914) centre (-0.8722, -21.8914) ccw
  arc A169 (2.0722, -21.8914) -> (0.8722, -20.6914) centre (0.8722, -21.8914) ccw
  arc A170 (0.8722, -28.9486) -> (2.0722, -27.7486) centre (0.8722, -27.7486) ccw
  arc A171 (-2.0722, -27.7486) -> (-0.8722, -28.9486) centre (-0.8722, -27.7486) ccw
  line L266 (-0.8722, -16.5386) -> (0.8722, -16.5386)
  line L267 (2.0722, -15.3386) -> (2.0722, -9.4814)
  line L268 (0.8722, -8.2814) -> (-0.8722, -8.2814)
  line L269 (-2.0722, -9.4814) -> (-2.0722, -15.3386)
  line L270 (-2.0722, -16.5386) -> (2.0722, -8.2814) construction
  line L271 (2.0722, -16.5386) -> (-2.0722, -8.2814) construction
  arc A172 (-0.8722, -8.2814) -> (-2.0722, -9.4814) centre (-0.8722, -9.4814) ccw
  arc A173 (2.0722, -9.4814) -> (0.8722, -8.2814) centre (0.8722, -9.4814) ccw
  arc A174 (0.8722, -16.5386) -> (2.0722, -15.3386) centre (0.8722, -15.3386) ccw
  arc A175 (-2.0722, -15.3386) -> (-0.8722, -16.5386) centre (-0.8722, -15.3386) ccw
  line L272 (-0.8722, -4.1286) -> (0.8722, -4.1286)
  line L273 (2.0722, -2.9286) -> (2.0722, 2.9286)
  line L274 (0.8722, 4.1286) -> (-0.8722, 4.1286)
  line L275 (-2.0722, 2.9286) -> (-2.0722, -2.9286)
  line L276 (-2.0722, -4.1286) -> (2.0722, 4.1286) construction
  line L277 (2.0722, -4.1286) -> (-2.0722, 4.1286) construction
  arc A176 (-0.8722, 4.1286) -> (-2.0722, 2.9286) centre (-0.8722, 2.9286) ccw
  arc A177 (2.0722, 2.9286) -> (0.8722, 4.1286) centre (0.8722, 2.9286) ccw
  arc A178 (0.8722, -4.1286) -> (2.0722, -2.9286) centre (0.8722, -2.9286) ccw
  arc A179 (-2.0722, -2.9286) -> (-0.8722, -4.1286) centre (-0.8722, -2.9286) ccw
  line L278 (-0.8722, 8.2814) -> (0.8722, 8.2814)
  line L279 (2.0722, 9.4814) -> (2.0722, 15.3386)
  line L280 (0.8722, 16.5386) -> (-0.8722, 16.5386)
  line L281 (-2.0722, 15.3386) -> (-2.0722, 9.4814)
  line L282 (-2.0722, 8.2814) -> (2.0722, 16.5386) construction
  line L283 (2.0722, 8.2814) -> (-2.0722, 16.5386) construction
  arc A180 (-0.8722, 16.5386) -> (-2.0722, 15.3386) centre (-0.8722, 15.3386) ccw
  arc A181 (2.0722, 15.3386) -> (0.8722, 16.5386) centre (0.8722, 15.3386) ccw
  arc A182 (0.8722, 8.2814) -> (2.0722, 9.4814) centre (0.8722, 9.4814) ccw
  arc A183 (-2.0722, 9.4814) -> (-0.8722, 8.2814) centre (-0.8722, 9.4814) ccw
  line L284 (-0.8722, 20.6914) -> (0.8722, 20.6914)
  line L285 (2.0722, 21.8914) -> (2.0722, 27.7486)
  line L286 (0.8722, 28.9486) -> (-0.8722, 28.9486)
  line L287 (-2.0722, 27.7486) -> (-2.0722, 21.8914)
  line L288 (-2.0722, 20.6914) -> (2.0722, 28.9486) construction
  line L289 (2.0722, 20.6914) -> (-2.0722, 28.9486) construction
  arc A184 (-0.8722, 28.9486) -> (-2.0722, 27.7486) centre (-0.8722, 27.7486) ccw
  arc A185 (2.0722, 27.7486) -> (0.8722, 28.9486) centre (0.8722, 27.7486) ccw
  arc A186 (0.8722, 20.6914) -> (2.0722, 21.8914) centre (0.8722, 21.8914) ccw
  arc A187 (-2.0722, 21.8914) -> (-0.8722, 20.6914) centre (-0.8722, 21.8914) ccw
  line L290 (-0.8722, -41.3586) -> (0.8722, -41.3586)
  line L291 (2.0722, -40.1586) -> (2.0722, -34.3014)
  line L292 (0.8722, -33.1014) -> (-0.8722, -33.1014)
  line L293 (-2.0722, -34.3014) -> (-2.0722, -40.1586)
  line L294 (-2.0722, -41.3586) -> (2.0722, -33.1014) construction
  line L295 (2.0722, -41.3586) -> (-2.0722, -33.1014) construction
  arc A188 (-0.8722, -33.1014) -> (-2.0722, -34.3014) centre (-0.8722, -34.3014) ccw
  arc A189 (2.0722, -34.3014) -> (0.8722, -33.1014) centre (0.8722, -34.3014) ccw
  arc A190 (0.8722, -41.3586) -> (2.0722, -40.1586) centre (0.8722, -40.1586) ccw
  arc A191 (-2.0722, -40.1586) -> (-0.8722, -41.3586) centre (-0.8722, -40.1586) ccw
  line L296 (-0.8722, -28.9486) -> (0.8722, -28.9486)
  line L297 (2.0722, -27.7486) -> (2.0722, -21.8914)
  line L298 (0.8722, -20.6914) -> (-0.8722, -20.6914)
  line L299 (-2.0722, -21.8914) -> (-2.0722, -27.7486)
  line L300 (-2.0722, -28.9486) -> (2.0722, -20.6914) construction
  line L301 (2.0722, -28.9486) -> (-2.0722, -20.6914) construction
  arc A192 (-0.8722, -20.6914) -> (-2.0722, -21.8914) centre (-0.8722, -21.8914) ccw
  arc A193 (2.0722, -21.8914) -> (0.8722, -20.6914) centre (0.8722, -21.8914) ccw
  arc A194 (0.8722, -28.9486) -> (2.0722, -27.7486) centre (0.8722, -27.7486) ccw
  arc A195 (-2.0722, -27.7486) -> (-0.8722, -28.9486) centre (-0.8722, -27.7486) ccw
  line L302 (-0.8722, -16.5386) -> (0.8722, -16.5386)
  line L303 (2.0722, -15.3386) -> (2.0722, -9.4814)
  line L304 (0.8722, -8.2814) -> (-0.8722, -8.2814)
  line L305 (-2.0722, -9.4814) -> (-2.0722, -15.3386)
  line L306 (-2.0722, -16.5386) -> (2.0722, -8.2814) construction
  line L307 (2.0722, -16.5386) -> (-2.0722, -8.2814) construction
  arc A196 (-0.8722, -8.2814) -> (-2.0722, -9.4814) centre (-0.8722, -9.4814) ccw
  arc A197 (2.0722, -9.4814) -> (0.8722, -8.2814) centre (0.8722, -9.4814) ccw
  arc A198 (0.8722, -16.5386) -> (2.0722, -15.3386) centre (0.8722, -15.3386) ccw
  arc A199 (-2.0722, -15.3386) -> (-0.8722, -16.5386) centre (-0.8722, -15.3386) ccw
  line L308 (-0.8722, -4.1286) -> (0.8722, -4.1286)
  line L309 (2.0722, -2.9286) -> (2.0722, 2.9286)
  line L310 (0.8722, 4.1286) -> (-0.8722, 4.1286)
  line L311 (-2.0722, 2.9286) -> (-2.0722, -2.9286)
  line L312 (-2.0722, -4.1286) -> (2.0722, 4.1286) construction
  line L313 (2.0722, -4.1286) -> (-2.0722, 4.1286) construction
  arc A200 (-0.8722, 4.1286) -> (-2.0722, 2.9286) centre (-0.8722, 2.9286) ccw
  arc A201 (2.0722, 2.9286) -> (0.8722, 4.1286) centre (0.8722, 2.9286) ccw
  arc A202 (0.8722, -4.1286) -> (2.0722, -2.9286) centre (0.8722, -2.9286) ccw
  arc A203 (-2.0722, -2.9286) -> (-0.8722, -4.1286) centre (-0.8722, -2.9286) ccw
  line L314 (-0.8722, 8.2814) -> (0.8722, 8.2814)
  line L315 (2.0722, 9.4814) -> (2.0722, 15.3386)
  line L316 (0.8722, 16.5386) -> (-0.8722, 16.5386)
  line L317 (-2.0722, 15.3386) -> (-2.0722, 9.4814)
  line L318 (-2.0722, 8.2814) -> (2.0722, 16.5386) construction
  line L319 (2.0722, 8.2814) -> (-2.0722, 16.5386) construction
  arc A204 (-0.8722, 16.5386) -> (-2.0722, 15.3386) centre (-0.8722, 15.3386) ccw
  arc A205 (2.0722, 15.3386) -> (0.8722, 16.5386) centre (0.8722, 15.3386) ccw
  arc A206 (0.8722, 8.2814) -> (2.0722, 9.4814) centre (0.8722, 9.4814) ccw
  arc A207 (-2.0722, 9.4814) -> (-0.8722, 8.2814) centre (-0.8722, 9.4814) ccw
  line L320 (-0.8722, -53.7686) -> (0.8722, -53.7686)
  line L321 (2.0722, -52.5686) -> (2.0722, -46.7114)
  line L322 (0.8722, -45.5114) -> (-0.8722, -45.5114)
  line L323 (-2.0722, -46.7114) -> (-2.0722, -52.5686)
  line L324 (-2.0722, -53.7686) -> (2.0722, -45.5114) construction
  line L325 (2.0722, -53.7686) -> (-2.0722, -45.5114) construction
  arc A208 (-0.8722, -45.5114) -> (-2.0722, -46.7114) centre (-0.8722, -46.7114) ccw
  arc A209 (2.0722, -46.7114) -> (0.8722, -45.5114) centre (0.8722, -46.7114) ccw
  arc A210 (0.8722, -53.7686) -> (2.0722, -52.5686) centre (0.8722, -52.5686) ccw
  arc A211 (-2.0722, -52.5686) -> (-0.8722, -53.7686) centre (-0.8722, -52.5686) ccw
  line L326 (-0.8722, -41.3586) -> (0.8722, -41.3586)
  line L327 (2.0722, -40.1586) -> (2.0722, -34.3014)
  line L328 (0.8722, -33.1014) -> (-0.8722, -33.1014)
  line L329 (-2.0722, -34.3014) -> (-2.0722, -40.1586)
  line L330 (-2.0722, -41.3586) -> (2.0722, -33.1014) construction
  line L331 (2.0722, -41.3586) -> (-2.0722, -33.1014) construction
  arc A212 (-0.8722, -33.1014) -> (-2.0722, -34.3014) centre (-0.8722, -34.3014) ccw
  arc A213 (2.0722, -34.3014) -> (0.8722, -33.1014) centre (0.8722, -34.3014) ccw
  arc A214 (0.8722, -41.3586) -> (2.0722, -40.1586) centre (0.8722, -40.1586) ccw
  arc A215 (-2.0722, -40.1586) -> (-0.8722, -41.3586) centre (-0.8722, -40.1586) ccw
  line L332 (-0.8722, -28.9486) -> (0.8722, -28.9486)
  line L333 (2.0722, -27.7486) -> (2.0722, -21.8914)
  line L334 (0.8722, -20.6914) -> (-0.8722, -20.6914)
  line L335 (-2.0722, -21.8914) -> (-2.0722, -27.7486)
  line L336 (-2.0722, -28.9486) -> (2.0722, -20.6914) construction
  line L337 (2.0722, -28.9486) -> (-2.0722, -20.6914) construction
  arc A216 (-0.8722, -20.6914) -> (-2.0722, -21.8914) centre (-0.8722, -21.8914) ccw
  arc A217 (2.0722, -21.8914) -> (0.8722, -20.6914) centre (0.8722, -21.8914) ccw
  arc A218 (0.8722, -28.9486) -> (2.0722, -27.7486) centre (0.8722, -27.7486) ccw
  arc A219 (-2.0722, -27.7486) -> (-0.8722, -28.9486) centre (-0.8722, -27.7486) ccw
  line L338 (-0.8722, -16.5386) -> (0.8722, -16.5386)
  line L339 (2.0722, -15.3386) -> (2.0722, -9.4814)
  line L340 (0.8722, -8.2814) -> (-0.8722, -8.2814)
  line L341 (-2.0722, -9.4814) -> (-2.0722, -15.3386)
  line L342 (-2.0722, -16.5386) -> (2.0722, -8.2814) construction
  line L343 (2.0722, -16.5386) -> (-2.0722, -8.2814) construction
  arc A220 (-0.8722, -8.2814) -> (-2.0722, -9.4814) centre (-0.8722, -9.4814) ccw
  arc A221 (2.0722, -9.4814) -> (0.8722, -8.2814) centre (0.8722, -9.4814) ccw
  arc A222 (0.8722, -16.5386) -> (2.0722, -15.3386) centre (0.8722, -15.3386) ccw
  arc A223 (-2.0722, -15.3386) -> (-0.8722, -16.5386) centre (-0.8722, -15.3386) ccw
  line L344 (-0.8722, -4.1286) -> (0.8722, -4.1286)
  line L345 (2.0722, -2.9286) -> (2.0722, 2.9286)
  line L346 (0.8722, 4.1286) -> (-0.8722, 4.1286)
  line L347 (-2.0722, 2.9286) -> (-2.0722, -2.9286)
  line L348 (-2.0722, -4.1286) -> (2.0722, 4.1286) construction
  line L349 (2.0722, -4.1286) -> (-2.0722, 4.1286) construction
  arc A224 (-0.8722, 4.1286) -> (-2.0722, 2.9286) centre (-0.8722, 2.9286) ccw
  arc A225 (2.0722, 2.9286) -> (0.8722, 4.1286) centre (0.8722, 2.9286) ccw
  arc A226 (0.8722, -4.1286) -> (2.0722, -2.9286) centre (0.8722, -2.9286) ccw
  arc A227 (-2.0722, -2.9286) -> (-0.8722, -4.1286) centre (-0.8722, -2.9286) ccw
  line L350 (-50.0055, -35.0091) -> (-50.0055, 35.0476) projected
  line L351 (-62.7055, -7.7) -> (-59.4055, -7.7)
  line L352 (-57.2055, -5.5) -> (-57.2055, 5.5)
  line L353 (-59.4055, 7.7) -> (-62.7055, 7.7)
  line L354 (-64.9055, 5.5) -> (-64.9055, -5.5)
  line L355 (-64.9055, -7.7) -> (-57.2055, 7.7) construction
  line L356 (-57.2055, -7.7) -> (-64.9055, 7.7) construction
  arc A228 (-62.7055, 7.7) -> (-64.9055, 5.5) centre (-62.7055, 5.5) ccw
  arc A229 (-57.2055, 5.5) -> (-59.4055, 7.7) centre (-59.4055, 5.5) ccw
  arc A230 (-59.4055, -7.7) -> (-57.2055, -5.5) centre (-59.4055, -5.5) ccw
  arc A231 (-64.9055, -5.5) -> (-62.7055, -7.7) centre (-62.7055, -5.5) ccw
  line L357 (-62.7055, 12.3) -> (-59.4055, 12.3)
  line L358 (-57.2055, 14.5) -> (-57.2055, 25.5)
  line L359 (-59.4055, 27.7) -> (-62.7055, 27.7)
  line L360 (-64.9055, 25.5) -> (-64.9055, 14.5)
  line L361 (-64.9055, 12.3) -> (-57.2055, 27.7) construction
  line L362 (-57.2055, 12.3) -> (-64.9055, 27.7) construction
  arc A232 (-62.7055, 27.7) -> (-64.9055, 25.5) centre (-62.7055, 25.5) ccw
  arc A233 (-57.2055, 25.5) -> (-59.4055, 27.7) centre (-59.4055, 25.5) ccw
  arc A234 (-59.4055, 12.3) -> (-57.2055, 14.5) centre (-59.4055, 14.5) ccw
  arc A235 (-64.9055, 14.5) -> (-62.7055, 12.3) centre (-62.7055, 14.5) ccw
  line L363 (-62.7055, -27.7) -> (-59.4055, -27.7)
  line L364 (-57.2055, -25.5) -> (-57.2055, -14.5)
  line L365 (-59.4055, -12.3) -> (-62.7055, -12.3)
  line L366 (-64.9055, -14.5) -> (-64.9055, -25.5)
  line L367 (-64.9055, -27.7) -> (-57.2055, -12.3) construction
  line L368 (-57.2055, -27.7) -> (-64.9055, -12.3) construction
  arc A236 (-62.7055, -12.3) -> (-64.9055, -14.5) centre (-62.7055, -14.5) ccw
  arc A237 (-57.2055, -14.5) -> (-59.4055, -12.3) centre (-59.4055, -14.5) ccw
  arc A238 (-59.4055, -27.7) -> (-57.2055, -25.5) centre (-59.4055, -25.5) ccw
  arc A239 (-64.9055, -25.5) -> (-62.7055, -27.7) centre (-62.7055, -25.5) ccw
  line L369 (-62.7055, -7.7) -> (-59.4055, -7.7)
  line L370 (-57.2055, -5.5) -> (-57.2055, 5.5)
  line L371 (-59.4055, 7.7) -> (-62.7055, 7.7)
  line L372 (-64.9055, 5.5) -> (-64.9055, -5.5)
  line L373 (-64.9055, -7.7) -> (-57.2055, 7.7) construction
  line L374 (-57.2055, -7.7) -> (-64.9055, 7.7) construction
  arc A240 (-62.7055, 7.7) -> (-64.9055, 5.5) centre (-62.7055, 5.5) ccw
  arc A241 (-57.2055, 5.5) -> (-59.4055, 7.7) centre (-59.4055, 5.5) ccw
  arc A242 (-59.4055, -7.7) -> (-57.2055, -5.5) centre (-59.4055, -5.5) ccw
  arc A243 (-64.9055, -5.5) -> (-62.7055, -7.7) centre (-62.7055, -5.5) ccw
  line L375 (-63.7413, -39.95) -> (-58.1413, -39.95)
  line L376 (-55.9413, -37.75) -> (-55.9413, -37.15)
  line L377 (-58.1413, -34.95) -> (-63.7413, -34.95)
  line L378 (-65.9413, -37.15) -> (-65.9413, -37.75)
  line L379 (-65.9413, -39.95) -> (-55.9413, -34.95) construction
  line L380 (-55.9413, -39.95) -> (-65.9413, -34.95) construction
  arc A244 (-63.7413, -34.95) -> (-65.9413, -37.15) centre (-63.7413, -37.15) ccw
  arc A245 (-65.9413, -37.75) -> (-63.7413, -39.95) centre (-63.7413, -37.75) ccw
  arc A246 (-58.1413, -39.95) -> (-55.9413, -37.75) centre (-58.1413, -37.75) ccw
  arc A247 (-55.9413, -37.15) -> (-58.1413, -34.95) centre (-58.1413, -37.15) ccw
  line L381 (-63.7413, 39.95) -> (-58.1413, 39.95)
  line L382 (-55.9413, 37.75) -> (-55.9413, 37.15)
  line L383 (-58.1413, 34.95) -> (-63.7413, 34.95)
  line L384 (-65.9413, 37.15) -> (-65.9413, 37.75)
  line L385 (-65.9413, 39.95) -> (-55.9413, 34.95) construction
  line L386 (-55.9413, 39.95) -> (-65.9413, 34.95) construction
  arc A248 (-65.9413, 37.15) -> (-63.7413, 34.95) centre (-63.7413, 37.15) ccw
  arc A249 (-63.7413, 39.95) -> (-65.9413, 37.75) centre (-63.7413, 37.75) ccw
  arc A250 (-55.9413, 37.75) -> (-58.1413, 39.95) centre (-58.1413, 37.75) ccw
  arc A251 (-58.1413, 34.95) -> (-55.9413, 37.15) centre (-58.1413, 37.15) ccw
  line L387 (71.9413, 0) -> (-71.9413, 0) construction
  line L388 (-71.9413, 0) -> (71.9413, 0) construction
  line L389 (62.7055, -7.7) -> (59.4055, -7.7)
  line L390 (57.2055, -5.5) -> (57.2055, 5.5)
  line L391 (59.4055, 7.7) -> (62.7055, 7.7)
  line L392 (64.9055, 5.5) -> (64.9055, -5.5)
  line L393 (64.9055, -7.7) -> (57.2055, 7.7) construction
  line L394 (57.2055, -7.7) -> (64.9055, 7.7) construction
  arc A252 (64.9055, 5.5) -> (62.7055, 7.7) centre (62.7055, 5.5) ccw
  arc A253 (59.4055, 7.7) -> (57.2055, 5.5) centre (59.4055, 5.5) ccw
  arc A254 (57.2055, -5.5) -> (59.4055, -7.7) centre (59.4055, -5.5) ccw
  arc A255 (62.7055, -7.7) -> (64.9055, -5.5) centre (62.7055, -5.5) ccw
  arc A256 (59.4055, 27.7) -> (57.2055, 25.5) centre (59.4055, 25.5) ccw
  line L395 (59.4055, 27.7) -> (62.7055, 27.7)
  arc A257 (64.9055, 25.5) -> (62.7055, 27.7) centre (62.7055, 25.5) ccw
  line L396 (57.2055, 14.5) -> (57.2055, 25.5)
  line L397 (62.7055, 12.3) -> (59.4055, 12.3)
  arc A258 (57.2055, 14.5) -> (59.4055, 12.3) centre (59.4055, 14.5) ccw
  line L398 (64.9055, 25.5) -> (64.9055, 14.5)
  line L399 (64.9055, 12.3) -> (57.2055, 27.7) construction
  line L400 (57.2055, 12.3) -> (64.9055, 27.7) construction